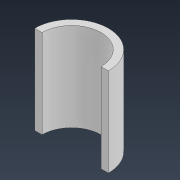
# Autodesk Inventor part: Panewka wałka rozrzadu srodek
Saved by Autodesk Inventor 2022 (Build 260153000, 153)
## iProperties
Created: 2023-05-22
Part Number: Panewka wałka rozrzadu srodek
Material: Generic
Document SubType Name: Modeling
Designer: wikto
Density: 1 g/cm^3
Appearance: Default
Author: wikto
Autodesk Inventor part; units mm, degrees
ref_plane "YZ Plane" through (0, 0, 0) normal (1, 0, 0) x (0, 1, 0)
ref_plane "XZ Plane" through (0, 0, 0) normal (0, 1, 0) x (-1, 0, 0)
ref_plane "XY Plane" through (0, 0, 0) normal (0, 0, 1) x (1, 0, 0)
sketch "Sketch1" plane through (0, 0, 0) normal (0, 1, 0) x (-1, 0, 0)
  arc A0 (-10, 0) -> (10, 0) centre (0, 0) ccw
  arc A1 (-12.5, 0) -> (12.5, 0) centre (0, 0) ccw
  line L0 (12.5, 0) -> (10, 0)
  line L1 (-10, 0) -> (-12.5, 0)
  line L2 (10, 0) -> (-10, 0)
  dimension "d0" = 20
  dimension "d1" = 25
  constraints: 6 end point, 4 point on circle, 3 horizontal, 2 centre point, 2 coincident, 2 horizontal alignment
  measures "d0" diameter of A0
  measures "d1" diameter of A1
extrude "Extrusion1" add sketch "Sketch1" along normal mid plane 30 contours A0 L0 A1 L1
body "Solid1"
